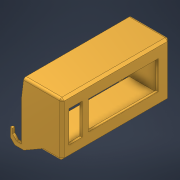
# Autodesk Inventor part: Mount Case
Saved by Autodesk Inventor 2022 (Build 260153000, 153)
## iProperties
Created: 2021-08-06
Part Number: Mount Case
Material: Generic
Document SubType Name: Modeling
Designer: sidsa
Density: 1 g/cm^3
Appearance: Brass - Satin
Author: sidsa
Autodesk Inventor part; units mm, degrees
ref_plane "YZ Plane" through (0, 0, 0) normal (1, 0, 0) x (0, 1, 0)
ref_plane "XZ Plane" through (0, 0, 0) normal (0, 1, 0) x (-1, 0, 0)
ref_plane "XY Plane" through (0, 0, 0) normal (0, 0, 1) x (1, 0, 0)
sketch "Sketch1" plane through (0, 0, 0) normal (1, 0, 0) x (0, 1, 0)
  line L0 (0, 0) -> (76.2, 0)
  line L1 (76.2, 0) -> (76.2, -152.4)
  line L2 (76.2, -152.4) -> (0, -152.4)
  line L3 (0, -152.4) -> (0, 0)
  line L4 (38.1, -152.4) -> (38.1, 0)
  line L5 (18.0975, -135.89) -> (18.0975, -38.1)
  line L6 (18.0975, -38.1) -> (58.1025, -38.1)
  line L7 (58.1025, -38.1) -> (58.1025, -135.89)
  line L8 (58.1025, -135.89) -> (18.0975, -135.89)
  line L9 (18.0975, -135.89) -> (58.1025, -38.1) construction
  line L10 (18.0975, -38.1) -> (58.1025, -135.89) construction
  point P0 (38.1, -86.995)
  dimension "d0" = 152.4
  dimension "d1" = 76.2
  dimension "d4" = 97.79
  dimension "d5" = 40.005
  dimension "d6" = 38.1
  constraints: 22 end point, 4 midpoint, 4 parallel, 2 perpendicular, 1 horizontal, 1 point on line
  measures "d0" distance of L0.end L1.end
  measures "d1" distance of L1.end L2.end
  measures "d4" distance of L5.start L5.end
  measures "d5" distance of L5.end L6.end
  measures "d6" distance between parallel lines of L0 L6
extrude "Extrusion1" add sketch "Sketch1" against normal blind 3.175 contours L0 L4 L6 L5 L8 L2 L3 | L0 L1 L2 L4 L8 L7 L6
sketch "Sketch2" plane through (-3.175, 0, 0) normal (-1, 0, 0) x (0, 0, 1)
  line L0 (-152.4, 0) -> (0, 0) projected
  line L1 (0, 0) -> (0, 76.2) projected
  line L2 (0, 76.2) -> (-152.4, 76.2) projected
  line L3 (-152.4, 76.2) -> (-152.4, 0) projected
  line L4 (-38.1, 58.1025) -> (-38.1, 18.0975) projected
  line L5 (-38.1, 18.0975) -> (-135.89, 18.0975) projected
  line L6 (-135.89, 18.0975) -> (-135.89, 58.1025) projected
  line L7 (-135.89, 58.1025) -> (-38.1, 58.1025) projected
  line L8 (-3.175, 73.025) -> (-3.175, 3.175)
  line L9 (-3.175, 3.175) -> (-149.225, 3.175)
  line L10 (-149.225, 3.175) -> (-149.225, 73.025)
  line L11 (-149.225, 73.025) -> (-3.175, 73.025)
  dimension "d9" = 3.175
  constraints: 8 end point, 3 other
  measures "d9" distance between parallel lines of L1 L8
extrude "Extrusion2" add sketch "Sketch2" along normal blind 50.8 contours L3 L2 L1 L0
sketch "Sketch3" plane through (0, 0, -152.4) normal (0, 0, -1) x (-1, 0, 0)
  line L0 (0, 0) -> (53.975, 0) projected
  line L1 (53.975, 0) -> (53.975, -12.7)
  line L2 (53.975, -12.7) -> (66.675, -12.7)
  line L3 (66.675, -12.7) -> (73.025, -6.35)
  line L4 (73.025, -6.35) -> (73.025, 6.35)
  line L5 (73.025, 6.35) -> (69.85, 6.35)
  line L6 (69.85, 6.35) -> (69.85, -0.5447)
  line L7 (69.85, -0.5447) -> (64.0447, -6.35)
  line L8 (64.0447, -6.35) -> (57.15, -6.35)
  line L9 (57.15, -6.35) -> (57.15, 0)
  line L10 (57.15, 0) -> (57.15, 50.8)
  line L11 (0, 76.2) -> (53.975, 76.2) projected
  line L12 (57.15, 50.8) -> (53.975, 76.2)
  line L13 (53.975, -12.7) -> (31.978, 0)
  line L14 (0, 0) -> (0, 76.2) projected
  line L15 (0, 0) -> (53.975, 0) projected
  line L16 (53.975, 76.2) -> (53.975, 0) projected
  line L17 (0, 76.2) -> (53.975, 76.2) projected
  dimension "d12" = 12.7
  dimension "d15" = 12.7
  dimension "d16" = 3.175
  dimension "d17" = 50.8
  dimension "d18" = 3.175
  dimension "d19" = 6.35
  dimension "d20" = 6.35
  dimension "d21" = 12.7
  dimension "d22" = 6.35
  dimension "d23" = 135
  dimension "d24" = 25.4
  constraints: 24 end point, 4 perpendicular, 2 parallel, 2 point on line, 2 vertical
  measures "d12" distance of L0.end L1.end
  measures "d15" distance of L3.end L4.end
  measures "d16" distance of L4.end L5.end
  measures "d17" distance of L9.end L10.end
  measures "d18" distance between parallel lines of L1 L9
  measures "d19" distance between parallel lines of L2 L8
  measures "d20" distance between parallel lines of L3 L7
  measures "d21" distance of L1.end L2.end
  measures "d22" horizontal distance of L2.end L3.end
  measures "d23" angle of L2 L3
  measures "d24" distance of L1.end L13.end
extrude "Extrusion3" add sketch "Sketch3" against normal blind 3.175 contours L0 L1 L13 | L16 L12 L10 L9 L8 L7 L6 L5 L4 L3 L2 L1
ref_plane "Work Plane1" through (0, 0, -76.2) normal (0, 0, -1) x (-1, 0, 0)
mirror "Mirror1" about plane through (0, 0, -76.2) normal (0, 0, -1) of "Extrusion3"
sketch "Sketch4" plane through (0, 0, -152.4) normal (0, 0, -1) x (-1, 0, 0)
  line L0 (0, 0) -> (0, 76.2) projected
  line L1 (0, 0) -> (31.978, 0) projected
  line L2 (31.978, 0) -> (53.975, -12.7) projected
  line L3 (53.975, -12.7) -> (66.675, -12.7) projected
  line L4 (66.675, -12.7) -> (73.025, -6.35) projected
  line L5 (73.025, -6.35) -> (73.025, 6.35) projected
  line L6 (73.025, 6.35) -> (69.85, 6.35) projected
  line L7 (69.85, 6.35) -> (69.85, -0.5447) projected
  line L8 (69.85, -0.5447) -> (64.0447, -6.35) projected
  line L9 (64.0447, -6.35) -> (57.15, -6.35) projected
  line L10 (57.15, -6.35) -> (57.15, 50.8) projected
  line L11 (57.15, 50.8) -> (53.975, 76.2) projected
  line L12 (0, 76.2) -> (53.975, 76.2) projected
  line L13 (7.62, 68.58) -> (7.62, 7.62)
  line L14 (7.62, 7.62) -> (34.0197, 7.62)
  line L15 (34.0197, 7.62) -> (49.53, -1.3349)
  line L16 (49.53, -1.3349) -> (49.53, 50.3256)
  line L17 (49.53, 50.3256) -> (47.2482, 68.58)
  line L18 (47.2482, 68.58) -> (7.62, 68.58)
  line L19 (49.53, 49.8475) -> (7.62, 49.8475)
  line L20 (10.4775, 49.8475) -> (10.4775, 68.58)
  point P0 (0, 0)
  dimension "d27" = 7.62
  constraints: 16 end point, 4 point on line, 2 perpendicular, 5 other
  measures "d27" distance between parallel lines of L0 L13
extrude "Extrusion4" cut sketch "Sketch4" against normal blind 3.175 contours L18 L20 L19 L13
fillet "Fillet1" radius 3.175 4 edges at (-15.989, 0, -152.4) (-15.989, 0, 0) (-26.9875, 76.2, -152.4) (-26.9875, 76.2, 0)
chamfer "Chamfer1" distance 0.3969 angle 45 4 edges at (0, 38.1, -38.1) (0, 18.0975, -86.995) (0, 58.1025, -86.995) (0, 38.1, -135.89)
chamfer "Chamfer2" distance 3.175 angle 45 8 edges at (0, 0, -76.2) (0, 0.9299, -151.4701) (0, 38.1, -152.4) (0, 75.2701, -151.4701) (0, 76.2, -76.2) (0, 75.2701, -0.9299) (0, 38.1, 0) (0, 0.9299, -0.9299)
pattern_linear "Rectangular Pattern1" count 5 spacing 9.525 along (-1, 0, 0) of "Extrusion4"
sketch "Sketch5" plane through (0, 0, 0) normal (1, 0, 0) x (0, 0, -1)
  line L0 (37.7031, 58.4994) -> (37.7031, 17.7006) projected
  line L1 (136.2869, 58.4994) -> (37.7031, 58.4994) projected
  line L2 (136.2869, 17.7006) -> (136.2869, 58.4994) projected
  line L3 (37.7031, 17.7006) -> (136.2869, 17.7006) projected
  line L4 (3.175, 3.175) -> (3.175, 73.025) projected
  line L5 (149.225, 3.175) -> (3.175, 3.175) projected
  line L6 (149.225, 73.025) -> (149.225, 3.175) projected
  line L7 (3.175, 73.025) -> (149.225, 73.025) projected
  line L8 (3.175, 3.175) -> (3.175, 73.025) projected
  line L9 (3.175, 38.1) -> (37.7031, 38.1)
  line L10 (9.525, 60.325) -> (9.525, 15.875)
  line L11 (9.525, 15.875) -> (28.575, 15.875)
  line L12 (28.575, 15.875) -> (28.575, 60.325)
  line L13 (28.575, 60.325) -> (9.525, 60.325)
  line L14 (9.525, 60.325) -> (28.575, 15.875) construction
  line L15 (9.525, 15.875) -> (28.575, 60.325) construction
  point P0 (0, 0)
  point P1 (19.05, 38.1)
  dimension "d40" = 44.45
  dimension "d41" = 19.05
  dimension "d44" = 6.35
  constraints: 14 end point, 4 midpoint, 2 parallel, 2 perpendicular, 1 point on line
  measures "d40" distance of L10.start L10.end
  measures "d41" distance of L10.end L11.end
  measures "d44" distance between parallel lines of L4 L10
extrude "Extrusion5" cut sketch "Sketch5" against normal blind 12.7 contours L10 L13 L12 L9 | L9 L12 L11 L10
body "Solid1"
